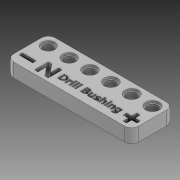
# Autodesk Inventor part: Drill Bushings Test Print
Saved by Autodesk Inventor 2022 (Build 260153000, 153)
## iProperties
Created: 2022-01-18
Part Number: Drill Bushings Test Print
Material: ABS Plastic
Document SubType Name: Modeling
Density: 1.06 g/cm^3
Appearance: Smooth - Medium Gray
Autodesk Inventor part; units mm, degrees
ref_plane "YZ Plane" through (0, 0, 0) normal (1, 0, 0) x (0, 1, 0)
ref_plane "XZ Plane" through (0, 0, 0) normal (0, 1, 0) x (-1, 0, 0)
ref_plane "XY Plane" through (0, 0, 0) normal (0, 0, 1) x (1, 0, 0)
sketch "Sketch1" plane through (0, 0, 0) normal (0, 1, 0) x (-1, 0, 0)
  line L0 (6.35, 20.6375) -> (-6.35, 20.6375)
  line L1 (-6.35, 20.6375) -> (-6.35, 17.4625)
  line L2 (-6.35, 17.4625) -> (6.35, 17.4625)
  line L3 (6.35, 17.4625) -> (6.35, 20.6375)
  line L4 (6.35, 20.6375) -> (-6.35, 17.4625) construction
  line L5 (-6.35, 20.6375) -> (6.35, 17.4625) construction
  line L6 (-88.9, 20.6375) -> (-101.6, 20.6375)
  line L7 (-101.6, 20.6375) -> (-101.6, 17.4625)
  line L8 (-101.6, 17.4625) -> (-88.9, 17.4625)
  line L9 (-88.9, 17.4625) -> (-88.9, 20.6375)
  line L10 (-88.9, 20.6375) -> (-101.6, 17.4625) construction
  line L11 (-101.6, 20.6375) -> (-88.9, 17.4625) construction
  line L12 (-96.8375, 12.7) -> (-93.6625, 12.7)
  line L13 (-93.6625, 12.7) -> (-93.6625, 25.4)
  line L14 (-93.6625, 25.4) -> (-96.8375, 25.4)
  line L15 (-96.8375, 25.4) -> (-96.8375, 12.7)
  line L16 (-96.8375, 12.7) -> (-93.6625, 25.4) construction
  line L17 (-93.6625, 12.7) -> (-96.8375, 25.4) construction
  line L18 (-12.7, 25.4) -> (-12.7, 12.7)
  line L19 (-12.7, 12.7) -> (-15.875, 12.7)
  line L20 (-15.875, 12.7) -> (-22.225, 20.407)
  line L21 (-22.225, 20.407) -> (-22.225, 12.7)
  line L22 (-22.225, 12.7) -> (-25.4, 12.7)
  line L23 (-25.4, 12.7) -> (-25.4, 25.4)
  line L24 (-25.4, 25.4) -> (-22.225, 25.4)
  line L25 (-22.225, 25.4) -> (-15.875, 17.693)
  line L26 (-15.875, 17.693) -> (-15.875, 25.4)
  line L27 (-15.875, 25.4) -> (-12.7, 25.4)
  line L28 (-19.05, 21.5465) -> (-19.05, 16.5535) construction
  line L29 (9.525, -9.525) -> (-104.775, -9.525)
  line L30 (-104.775, -9.525) -> (-104.775, 28.575)
  line L31 (-104.775, 28.575) -> (9.525, 28.575)
  line L32 (9.525, 28.575) -> (9.525, -9.525)
  line L33 (9.525, -9.525) -> (-104.775, 28.575) construction
  line L34 (-104.775, -9.525) -> (9.525, 28.575) construction
  line L35 (-28.7089, 13.4715) -> (-85.5911, 13.4715) construction
  line L36 (-85.5911, 13.4715) -> (-85.5911, 24.6285) construction
  line L37 (-85.5911, 24.6285) -> (-28.7089, 24.6285) construction
  line L38 (-28.7089, 24.6285) -> (-28.7089, 13.4715) construction
  spline S0 degree 2 poles (-35.3547, 18.2987) (-35.3547, 19.1889) (-34.5777, 20.5886) (-33.9859, 20.9643) knots 0 0 0 1 2 2 2
  spline S1 degree 2 poles (-33.9859, 20.9643) (-33.4919, 21.2833) (-32.3289, 21.4686) (-31.6754, 21.4686) knots 0 0 0 1 2 2 2
  line L39 (-31.6754, 21.4686) -> (-29.6891, 21.4686)
  line L40 (-29.6891, 21.4686) -> (-29.6891, 15.1186)
  line L41 (-29.6891, 15.1186) -> (-31.6548, 15.1186)
  spline S2 degree 2 poles (-31.6548, 15.1186) (-32.3238, 15.1186) (-33.4919, 15.2884) (-34.0065, 15.6177) knots 0 0 0 1 2 2 2
  spline S3 degree 2 poles (-34.0065, 15.6177) (-34.6291, 16.0191) (-35.3547, 17.3776) (-35.3547, 18.2987) knots 0 0 0 1 2 2 2
  spline S4 degree 2 poles (-33.7183, 18.2884) (-33.7183, 17.6606) (-33.286, 16.7652) (-32.8435, 16.5131) knots 0 0 0 1 2 2 2
  spline S5 degree 2 poles (-32.8435, 16.5131) (-32.5193, 16.3381) (-31.8092, 16.3021) (-31.3152, 16.3021) knots 0 0 0 1 2 2 2
  line L42 (-31.3152, 16.3021) -> (-31.2843, 16.3021)
  line L43 (-31.2843, 16.3021) -> (-31.2843, 20.2799)
  line L44 (-31.2843, 20.2799) -> (-31.3152, 20.2799)
  spline S6 degree 2 poles (-31.3152, 20.2799) (-31.8503, 20.2799) (-32.5862, 20.2438) (-32.9207, 20.0329) knots 0 0 0 1 2 2 2
  spline S7 degree 2 poles (-32.9207, 20.0329) (-33.3118, 19.7859) (-33.7183, 18.9162) (-33.7183, 18.2884) knots 0 0 0 1 2 2 2
  line L45 (-39.4302, 18.0929) -> (-39.3067, 18.0929)
  spline S8 degree 2 poles (-39.3067, 18.0929) (-39.2192, 18.062) (-38.895, 18.0311) (-38.6995, 18.0311) knots 0 0 0 1 2 2 2
  spline S9 degree 2 poles (-38.6995, 18.0311) (-38.4679, 18.0311) (-37.9482, 18.1701) (-37.7063, 18.2627) knots 0 0 0 1 2 2 2
  line L46 (-37.7063, 18.2627) -> (-37.7063, 21.4686)
  line L47 (-37.7063, 21.4686) -> (-36.214, 21.4686)
  line L48 (-36.214, 21.4686) -> (-36.214, 16.6778)
  line L49 (-36.214, 16.6778) -> (-37.7063, 16.6778)
  line L50 (-37.7063, 16.6778) -> (-37.7063, 17.3673)
  spline S10 degree 2 poles (-37.7063, 17.3673) (-37.8093, 17.2747) (-38.1695, 16.9865) (-38.3187, 16.899) knots 0 0 0 1 2 2 2
  spline S11 degree 2 poles (-38.3187, 16.899) (-38.4834, 16.8013) (-38.9156, 16.6623) (-39.106, 16.6623) knots 0 0 0 1 2 2 2
  spline S12 degree 2 poles (-39.106, 16.6623) (-39.1781, 16.6623) (-39.3582, 16.6726) (-39.4302, 16.6778) knots 0 0 0 1 2 2 2
  line L51 (-39.4302, 16.6778) -> (-39.4302, 18.0929)
  line L52 (-41.4937, 21.4686) -> (-40.0014, 21.4686)
  line L53 (-40.0014, 21.4686) -> (-40.0014, 16.6778)
  line L54 (-40.0014, 16.6778) -> (-41.4937, 16.6778)
  line L55 (-41.4937, 16.6778) -> (-41.4937, 21.4686)
  line L56 (-41.54, 15.9934) -> (-39.9602, 15.9934)
  line L57 (-39.9602, 15.9934) -> (-39.9602, 14.8304)
  line L58 (-39.9602, 14.8304) -> (-41.54, 14.8304)
  line L59 (-41.54, 14.8304) -> (-41.54, 15.9934)
  line L60 (-44.1284, 21.4686) -> (-42.6361, 21.4686)
  line L61 (-42.6361, 21.4686) -> (-42.6361, 14.8355)
  line L62 (-42.6361, 14.8355) -> (-44.1284, 14.8355)
  line L63 (-44.1284, 14.8355) -> (-44.1284, 21.4686)
  line L64 (-46.7631, 21.4686) -> (-45.2708, 21.4686)
  line L65 (-45.2708, 21.4686) -> (-45.2708, 14.8355)
  line L66 (-45.2708, 14.8355) -> (-46.7631, 14.8355)
  line L67 (-46.7631, 14.8355) -> (-46.7631, 21.4686)
  spline S13 degree 2 poles (-55.6243, 19.5234) (-55.6243, 19.9968) (-55.264, 20.7121) (-54.9656, 20.9488) knots 0 0 0 1 2 2 2
  spline S14 degree 2 poles (-54.9656, 20.9488) (-54.6054, 21.2318) (-53.7512, 21.4686) (-53.0873, 21.4686) knots 0 0 0 1 2 2 2
  line L68 (-53.0873, 21.4686) -> (-50.5504, 21.4686)
  line L69 (-50.5504, 21.4686) -> (-50.5504, 15.1186)
  line L70 (-50.5504, 15.1186) -> (-52.7889, 15.1186)
  spline S15 degree 2 poles (-52.7889, 15.1186) (-53.4887, 15.1186) (-54.2091, 15.2266) (-54.523, 15.3964) knots 0 0 0 1 2 2 2
  spline S16 degree 2 poles (-54.523, 15.3964) (-54.8678, 15.5765) (-55.2023, 16.194) (-55.2023, 16.5954) knots 0 0 0 1 2 2 2
  spline S17 degree 2 poles (-55.2023, 16.5954) (-55.2023, 17.0585) (-54.7392, 17.7841) (-54.3275, 17.9539) knots 0 0 0 1 2 2 2
  line L71 (-54.3275, 17.9539) -> (-54.3275, 17.9848)
  spline S18 degree 2 poles (-54.3275, 17.9848) (-54.9193, 18.1083) (-55.6243, 18.875) (-55.6243, 19.5234) knots 0 0 0 1 2 2 2
  spline S19 degree 2 poles (-53.9776, 19.4977) (-53.9776, 19.1992) (-53.7409, 18.8647) (-53.5042, 18.7773) knots 0 0 0 1 2 2 2
  spline S20 degree 2 poles (-53.5042, 18.7773) (-53.3601, 18.7207) (-52.8506, 18.7104) (-52.4287, 18.7104) knots 0 0 0 1 2 2 2
  line L72 (-52.4287, 18.7104) -> (-52.1354, 18.7104)
  line L73 (-52.1354, 18.7104) -> (-52.1354, 20.3107)
  line L74 (-52.1354, 20.3107) -> (-52.2228, 20.3107)
  spline S21 degree 2 poles (-52.2228, 20.3107) (-52.8403, 20.3107) (-53.3138, 20.2953) (-53.5608, 20.1872) knots 0 0 0 1 2 2 2
  spline S22 degree 2 poles (-53.5608, 20.1872) (-53.7769, 20.0895) (-53.9776, 19.7293) (-53.9776, 19.4977) knots 0 0 0 1 2 2 2
  spline S23 degree 2 poles (-53.5813, 16.9093) (-53.5813, 16.7549) (-53.4218, 16.4308) (-53.2572, 16.3587) knots 0 0 0 1 2 2 2
  spline S24 degree 2 poles (-53.2572, 16.3587) (-53.1028, 16.2867) (-52.6705, 16.2764) (-52.2434, 16.2764) knots 0 0 0 1 2 2 2
  line L75 (-52.2434, 16.2764) -> (-52.1354, 16.2764)
  line L76 (-52.1354, 16.2764) -> (-52.1354, 17.6246)
  line L77 (-52.1354, 17.6246) -> (-52.336, 17.6246)
  spline S25 degree 2 poles (-52.336, 17.6246) (-52.7426, 17.6246) (-53.0719, 17.6092) (-53.2469, 17.5268) knots 0 0 0 1 2 2 2
  spline S26 degree 2 poles (-53.2469, 17.5268) (-53.4373, 17.4342) (-53.5813, 17.1203) (-53.5813, 16.9093) knots 0 0 0 1 2 2 2
  line L78 (-60.8988, 21.4686) -> (-59.4065, 21.4686)
  line L79 (-59.4065, 21.4686) -> (-59.4065, 20.9385)
  spline S27 degree 2 poles (-59.4065, 20.9385) (-59.0205, 21.2627) (-58.3721, 21.6023) (-57.9245, 21.6023) knots 0 0 0 1 2 2 2
  spline S28 degree 2 poles (-57.9245, 21.6023) (-57.2143, 21.6023) (-56.4167, 20.7018) (-56.4167, 19.7962) knots 0 0 0 1 2 2 2
  line L80 (-56.4167, 19.7962) -> (-56.4167, 16.6778)
  line L81 (-56.4167, 16.6778) -> (-57.9193, 16.6778)
  line L82 (-57.9193, 16.6778) -> (-57.9193, 19.0551)
  spline S29 degree 2 poles (-57.9193, 19.0551) (-57.9193, 19.4256) (-57.9553, 19.8991) (-58.0274, 20.0586) knots 0 0 0 1 2 2 2
  spline S30 degree 2 poles (-58.0274, 20.0586) (-58.0994, 20.2078) (-58.3824, 20.3622) (-58.6397, 20.3622) knots 0 0 0 1 2 2 2
  spline S31 degree 2 poles (-58.6397, 20.3622) (-58.7941, 20.3622) (-59.2264, 20.2078) (-59.4065, 20.074) knots 0 0 0 1 2 2 2
  line L83 (-59.4065, 20.074) -> (-59.4065, 16.6778)
  line L84 (-59.4065, 16.6778) -> (-60.8988, 16.6778)
  line L85 (-60.8988, 16.6778) -> (-60.8988, 21.4686)
  spline S32 degree 2 poles (-63.4974, 21.5972) (-62.9725, 21.5972) (-62.0309, 21.3656) (-61.7221, 21.2113) knots 0 0 0 1 2 2 2
  line L86 (-61.7221, 21.2113) -> (-61.7221, 19.9505)
  line L87 (-61.7221, 19.9505) -> (-61.8456, 19.9505)
  spline S33 degree 2 poles (-61.8456, 19.9505) (-61.9537, 20.0329) (-62.2264, 20.2284) (-62.4683, 20.3365) knots 0 0 0 1 2 2 2
  spline S34 degree 2 poles (-62.4683, 20.3365) (-62.6792, 20.4342) (-63.199, 20.5732) (-63.5077, 20.5732) knots 0 0 0 1 2 2 2
  spline S35 degree 2 poles (-63.5077, 20.5732) (-63.8216, 20.5732) (-64.3053, 20.3776) (-64.3053, 20.1667) knots 0 0 0 1 2 2 2
  spline S36 degree 2 poles (-64.3053, 20.1667) (-64.3053, 20.002) (-64.0841, 19.827) (-63.765, 19.755) knots 0 0 0 1 2 2 2
  spline S37 degree 2 poles (-63.765, 19.755) (-63.5952, 19.7087) (-63.0755, 19.6109) (-62.8748, 19.5491) knots 0 0 0 1 2 2 2
  spline S38 degree 2 poles (-62.8748, 19.5491) (-62.3087, 19.3742) (-61.7427, 18.6898) (-61.7427, 18.1289) knots 0 0 0 1 2 2 2
  spline S39 degree 2 poles (-61.7427, 18.1289) (-61.7427, 17.8098) (-62.036, 17.2438) (-62.3242, 17.0225) knots 0 0 0 1 2 2 2
  spline S40 degree 2 poles (-62.3242, 17.0225) (-62.6072, 16.8064) (-63.446, 16.5491) (-63.976, 16.5491) knots 0 0 0 1 2 2 2
  spline S41 degree 2 poles (-63.976, 16.5491) (-64.4803, 16.5491) (-65.3242, 16.7498) (-65.6124, 16.8887) knots 0 0 0 1 2 2 2
  line L88 (-65.6124, 16.8887) -> (-65.6124, 18.1032)
  line L89 (-65.6124, 18.1032) -> (-65.494, 18.1032)
  spline S42 degree 2 poles (-65.494, 18.1032) (-65.4168, 18.0414) (-65.0824, 17.8407) (-64.928, 17.7687) knots 0 0 0 1 2 2 2
  spline S43 degree 2 poles (-64.928, 17.7687) (-64.7376, 17.6863) (-64.2745, 17.5731) (-64.0326, 17.5731) knots 0 0 0 1 2 2 2
  spline S44 degree 2 poles (-64.0326, 17.5731) (-63.7084, 17.5731) (-63.2607, 17.7944) (-63.2607, 17.9745) knots 0 0 0 1 2 2 2
  spline S45 degree 2 poles (-63.2607, 17.9745) (-63.2607, 18.1392) (-63.482, 18.3244) (-63.8525, 18.4171) knots 0 0 0 1 2 2 2
  spline S46 degree 2 poles (-63.8525, 18.4171) (-64.0429, 18.4634) (-64.542, 18.5509) (-64.7736, 18.628) knots 0 0 0 1 2 2 2
  spline S47 degree 2 poles (-64.7736, 18.628) (-65.2882, 18.7927) (-65.8234, 19.4359) (-65.8234, 19.9711) knots 0 0 0 1 2 2 2
  spline S48 degree 2 poles (-65.8234, 19.9711) (-65.8234, 20.3056) (-65.5095, 20.9179) (-65.2161, 21.1238) knots 0 0 0 1 2 2 2
  spline S49 degree 2 poles (-65.2161, 21.1238) (-64.9125, 21.3502) (-64.0789, 21.5972) (-63.4974, 21.5972) knots 0 0 0 1 2 2 2
  line L90 (-71.0155, 21.4686) -> (-69.5129, 21.4686)
  line L91 (-69.5129, 21.4686) -> (-69.5129, 19.0963)
  spline S50 degree 2 poles (-69.5129, 19.0963) (-69.5129, 18.803) (-69.4666, 18.2267) (-69.4049, 18.0929) knots 0 0 0 1 2 2 2
  spline S51 degree 2 poles (-69.4049, 18.0929) (-69.3277, 17.9282) (-69.0395, 17.7893) (-68.7925, 17.7893) knots 0 0 0 1 2 2 2
  spline S52 degree 2 poles (-68.7925, 17.7893) (-68.6124, 17.7893) (-68.2368, 17.9282) (-68.0258, 18.0774) knots 0 0 0 1 2 2 2
  line L92 (-68.0258, 18.0774) -> (-68.0258, 21.4686)
  line L93 (-68.0258, 21.4686) -> (-66.5335, 21.4686)
  line L94 (-66.5335, 21.4686) -> (-66.5335, 14.8355)
  line L95 (-66.5335, 14.8355) -> (-68.0258, 14.8355)
  line L96 (-68.0258, 14.8355) -> (-68.0258, 17.2078)
  spline S53 degree 2 poles (-68.0258, 17.2078) (-68.3911, 16.899) (-69.0858, 16.5491) (-69.5078, 16.5491) knots 0 0 0 1 2 2 2
  spline S54 degree 2 poles (-69.5078, 16.5491) (-70.2385, 16.5491) (-71.0155, 17.4754) (-71.0155, 18.3502) knots 0 0 0 1 2 2 2
  line L97 (-71.0155, 18.3502) -> (-71.0155, 21.4686)
  line L98 (-73.6142, 21.4686) -> (-72.1219, 21.4686)
  line L99 (-72.1219, 21.4686) -> (-72.1219, 16.6778)
  line L100 (-72.1219, 16.6778) -> (-73.6142, 16.6778)
  line L101 (-73.6142, 16.6778) -> (-73.6142, 21.4686)
  line L102 (-73.6605, 15.9934) -> (-72.0807, 15.9934)
  line L103 (-72.0807, 15.9934) -> (-72.0807, 14.8304)
  line L104 (-72.0807, 14.8304) -> (-73.6605, 14.8304)
  line L105 (-73.6605, 14.8304) -> (-73.6605, 15.9934)
  line L106 (-79.2386, 21.4686) -> (-77.736, 21.4686)
  line L107 (-77.736, 21.4686) -> (-77.736, 19.0963)
  spline S55 degree 2 poles (-77.736, 19.0963) (-77.736, 18.803) (-77.6897, 18.2267) (-77.628, 18.0929) knots 0 0 0 1 2 2 2
  spline S56 degree 2 poles (-77.628, 18.0929) (-77.5508, 17.9282) (-77.2626, 17.7893) (-77.0156, 17.7893) knots 0 0 0 1 2 2 2
  spline S57 degree 2 poles (-77.0156, 17.7893) (-76.8355, 17.7893) (-76.4599, 17.9282) (-76.2489, 18.0774) knots 0 0 0 1 2 2 2
  line L108 (-76.2489, 18.0774) -> (-76.2489, 21.4686)
  line L109 (-76.2489, 21.4686) -> (-74.7566, 21.4686)
  line L110 (-74.7566, 21.4686) -> (-74.7566, 16.6778)
  line L111 (-74.7566, 16.6778) -> (-76.2489, 16.6778)
  line L112 (-76.2489, 16.6778) -> (-76.2489, 17.2078)
  spline S58 degree 2 poles (-76.2489, 17.2078) (-76.6142, 16.899) (-77.3089, 16.5491) (-77.7309, 16.5491) knots 0 0 0 1 2 2 2
  spline S59 degree 2 poles (-77.7309, 16.5491) (-78.4616, 16.5491) (-79.2386, 17.4754) (-79.2386, 18.3502) knots 0 0 0 1 2 2 2
  line L113 (-79.2386, 18.3502) -> (-79.2386, 21.4686)
  spline S60 degree 2 poles (-84.6984, 20.9179) (-84.6984, 21.5818) (-84.3125, 22.5132) (-83.9831, 22.7705) knots 0 0 0 1 2 2 2
  spline S61 degree 2 poles (-83.9831, 22.7705) (-83.6486, 23.0329) (-82.7224, 23.2696) (-82.1563, 23.2696) knots 0 0 0 1 2 2 2
  spline S62 degree 2 poles (-82.1563, 23.2696) (-81.6778, 23.2696) (-80.8184, 23.1461) (-80.5045, 23.0638) knots 0 0 0 1 2 2 2
  line L114 (-80.5045, 23.0638) -> (-80.5045, 21.8648)
  line L115 (-80.5045, 21.8648) -> (-80.6795, 21.8648)
  spline S63 degree 2 poles (-80.6795, 21.8648) (-80.7875, 21.906) (-81.0911, 22.0089) (-81.2455, 22.05) knots 0 0 0 1 2 2 2
  spline S64 degree 2 poles (-81.2455, 22.05) (-81.4308, 22.0964) (-81.7807, 22.1581) (-81.9608, 22.1581) knots 0 0 0 1 2 2 2
  spline S65 degree 2 poles (-81.9608, 22.1581) (-82.3416, 22.1581) (-82.8459, 22.0037) (-82.9745, 21.8596) knots 0 0 0 1 2 2 2
  spline S66 degree 2 poles (-82.9745, 21.8596) (-83.1032, 21.7104) (-83.2061, 21.309) (-83.2061, 21.0003) knots 0 0 0 1 2 2 2
  line L116 (-83.2061, 21.0003) -> (-83.2061, 20.9128)
  spline S67 degree 2 poles (-83.2061, 20.9128) (-82.954, 21.1341) (-82.2953, 21.4017) (-81.9454, 21.4017) knots 0 0 0 1 2 2 2
  spline S68 degree 2 poles (-81.9454, 21.4017) (-81.014, 21.4017) (-80.0054, 20.1924) (-80.0054, 18.9522) knots 0 0 0 1 2 2 2
  spline S69 degree 2 poles (-80.0054, 18.9522) (-80.0054, 18.3913) (-80.3141, 17.4959) (-80.592, 17.1821) knots 0 0 0 1 2 2 2
  spline S70 degree 2 poles (-80.592, 17.1821) (-80.8596, 16.8784) (-81.6057, 16.5491) (-82.0123, 16.5491) knots 0 0 0 1 2 2 2
  spline S71 degree 2 poles (-82.0123, 16.5491) (-82.3776, 16.5491) (-82.9591, 16.7344) (-83.1958, 16.8887) knots 0 0 0 1 2 2 2
  line L117 (-83.1958, 16.8887) -> (-83.2524, 16.6778)
  line L118 (-83.2524, 16.6778) -> (-84.6984, 16.6778)
  line L119 (-84.6984, 16.6778) -> (-84.6984, 20.9179)
  line L120 (-83.2061, 19.9608) -> (-83.2061, 17.7893)
  spline S72 degree 2 poles (-83.2061, 17.7893) (-83.098, 17.7378) (-82.7738, 17.6709) (-82.6092, 17.6709) knots 0 0 0 1 2 2 2
  spline S73 degree 2 poles (-82.6092, 17.6709) (-82.074, 17.6709) (-81.5337, 18.3656) (-81.5337, 18.9882) knots 0 0 0 1 2 2 2
  spline S74 degree 2 poles (-81.5337, 18.9882) (-81.5337, 19.297) (-81.616, 19.7293) (-81.7241, 19.8939) knots 0 0 0 1 2 2 2
  spline S75 degree 2 poles (-81.7241, 19.8939) (-81.8322, 20.0586) (-82.1769, 20.2233) (-82.4445, 20.2233) knots 0 0 0 1 2 2 2
  spline S76 degree 2 poles (-82.4445, 20.2233) (-82.6452, 20.2233) (-83.0311, 20.0843) (-83.2061, 19.9608) knots 0 0 0 1 2 2 2
  point P0 (0, 19.05)
  point P1 (-95.25, 19.05)
  point P2 (-95.25, 19.05)
  point P3 (0, 19.05)
  point P4 (-95.25, 19.05)
  point P5 (0, 19.05)
  point P6 (-95.25, 19.05)
  point P7 (-96.8375, 20.6375)
  point P8 (-93.6625, 20.6375)
  point P9 (-93.6625, 17.4625)
  point P10 (-96.8375, 17.4625)
  point P11 (0, 0)
  point P12 (-19.05, 19.05)
  point P13 (-95.25, 19.05)
  point P14 (-19.05, 0)
  point P15 (-38.1, 0)
  point P16 (-57.15, 0)
  point P17 (-76.2, 0)
  point P18 (-47.625, 9.525)
  point P19 (-95.25, 0)
  point P20 (-28.7089, 19.05)
  point P21 (-57.15, 13.4715)
  dimension "d33" = 12.7
  dimension "d34" = 3.175
  dimension "d61" = 12.7
  dimension "d62" = 12.7
  dimension "d64" = 3.175
  dimension "d66" = 38.1
  dimension "d67" = 114.3
  dimension "d81" = 19.05
  dimension "d86" = 19.05
  dimension "d87" = 9.525
  dimension "d123" = 9.525
  constraints: 71 end point, 18 midpoint, 11 parallel, 7 equal length, 7 perpendicular, 6 point on line, 5 horizontal, 5 vertical alignment, 3 horizontal alignment, 1 vertical, 7 other
  measures "d33" distance of L1.end L2.end
  measures "d34" distance of L2.end L0.start
  measures "d61" distance between parallel lines of L23 L18
  measures "d62" distance between parallel lines of L24 L22
  measures "d64" distance between parallel lines of L25 L20
  measures "d66" distance of L29.end L30.end
  measures "d67" distance of L29.start L29.end
  measures "d81" distance of point (0, 0) point (-19.05, 0)
  measures "d86" distance of point (0, 19.05) point (0, 0)
  measures "d87" vertical distance of point (-47.625, 9.525) point (0, 19.05)
  measures "d123" horizontal distance of point (-47.625, 9.525) point (-38.1, 0)
extrude "Extrusion1" add sketch "Sketch1" against normal blind 12.7 contours L29 L30 L31 L32 | S0 S1 L39 L40 L41 S2 S3 | S7 S6 L44 L43 L42 S5 S4 | L45 S8 S9 L46 L47 L48 L49 L50 S10 S11 S12 L51 | L52 L53 L54 L55 | L56 L57 L58 L59 | L60 L61 L62 L63 | L64 L65 L66 L67 | S13 S14 L68 L69 L70 S15 S16 S17 L71 S18 | S22 S21 L74 L73 L72 S20 S19 | S26 S25 L77 L76 L75 S24 S23 | L78 L79 S27 S28 L80 L81 L82 S29 S30 S31 L83 L84 L85 | S32 L86 L87 S33 S34 S35 S36 S37 S38 S39 S40 S41 L88 L89 S42 S43 S44 S45 S46 S47 S48 S49 | L90 L91 S50 S51 S52 L92 L93 L94 L95 L96 S53 S54 L97 | L98 L99 L100 L101 | L102 L103 L104 L105 | L106 L107 S55 S56 S57 L108 L109 L110 L111 L112 S58 S59 L113 | S60 S61 S62 L114 L115 S63 S64 S65 S66 L116 S67 S68 S69 S70 S71 L117 L118 L119 | S76 S75 S74 S73 S72 L120
fillet "Fillet1" radius 6.35 4 edges at (-9.525, -6.35, 28.575) (-9.525, -6.35, -9.525) (104.775, -6.35, -9.525) (104.775, -6.35, 28.575)
fillet "Fillet2" radius 0.3969 26 edges at (22.225, -6.35, 20.407) (101.6, -6.35, 17.4625) (101.6, -6.35, 20.6375) (96.8375, -6.35, 20.6375) (96.8375, -6.35, 25.4) (93.6625, -6.35, 25.4) (93.6625, -6.35, 20.6375) (88.9, -6.35, 20.6375) (88.9, -6.35, 17.4625) (93.6625, -6.35, 17.4625) (93.6625, -6.35, 12.7) (96.8375, -6.35, 12.7) (96.8375, -6.35, 17.4625) (22.225, -6.35, 12.7) (25.4, -6.35, 12.7) (25.4, -6.35, 25.4) (22.225, -6.35, 25.4) (15.875, -6.35, 17.693) (15.875, -6.35, 12.7) (12.7, -6.35, 12.7) (15.875, -6.35, 25.4) (12.7, -6.35, 25.4) (6.35, -6.35, 20.6375) (6.35, -6.35, 17.4625) (-6.35, -6.35, 17.4625) (-6.35, -6.35, 20.6375)
hole "Hole1" at (19.05, 0, 0) direction (0, -1, 0) diameter 9.525 depth 12.7 counterbore diameter 11.9888 counterbore depth 1.905
hole "Hole2" at (0, 0, 0) direction (0, -1, 0) diameter 9.398 depth 12.7 counterbore diameter 11.8618 counterbore depth 1.905
hole "Hole3" at (38.1, 0, 0) direction (0, -1, 0) diameter 9.652 depth 12.7 counterbore diameter 12.1158 counterbore depth 1.905
hole "Hole4" at (57.15, 0, 0) direction (0, -1, 0) diameter 9.779 depth 12.7 counterbore diameter 12.2428 counterbore depth 1.905
hole "Hole5" at (76.2, 0, 0) direction (0, -1, 0) diameter 9.906 depth 12.7 counterbore diameter 12.3698 counterbore depth 1.905
hole "Hole6" at (95.25, 0, 0) direction (0, -1, 0) diameter 10.033 depth 12.7 counterbore diameter 12.4968 counterbore depth 1.905
emboss "Emboss1" sketch "Sketch1" operation cut depth 3.175 direction (0, -1, 0) contours S0 S1 L39 L40 L41 S2 S3 | L45 S8 S9 L46 L47 L48 L49 L50 S10 S11 S12 L51 | L52 L53 L54 L55 | L56 L57 L58 L59 | L60 L61 L62 L63 | L64 L65 L66 L67 | S13 S14 L68 L69 L70 S15 S16 S17 L71 S18 | L78 L79 S27 S28 L80 L81 L82 S29 S30 S31 L83 L84 L85 | S32 L86 L87 S33 S34 S35 S36 S37 S38 S39 S40 S41 L88 L89 S42 S43 S44 S45 S46 S47 S48 S49 | L90 L91 S50 S51 S52 L92 L93 L94 L95 L96 S53 S54 L97 | L98 L99 L100 L101 | L102 L103 L104 L105 | L106 L107 S55 S56 S57 L108 L109 L110 L111 L112 S58 S59 L113 | S60 S61 S62 L114 L115 S63 S64 S65 S66 L116 S67 S68 S69 S70 S71 L117 L118 L119
body "Solid1"
